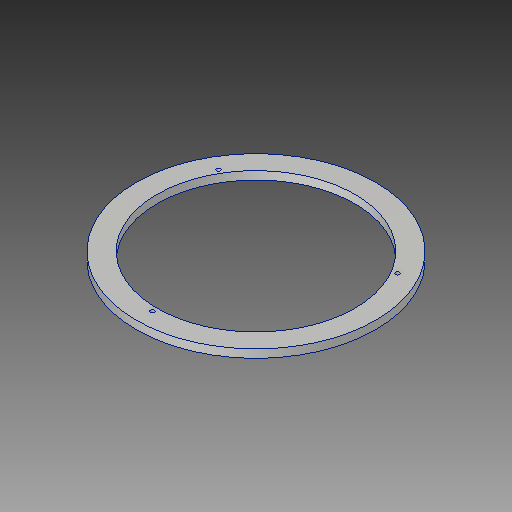
# Autodesk Inventor part: LazySusan
Saved by Autodesk Inventor 2019 (Build 230136000, 136)
## iProperties
Created: 2015-11-16
Part Number: LazySusan
Material: Aluminum 6061
Document SubType Name: Modeling
Designer: Vervaeke-Lab
Density: 2.7 g/cm^3
Appearance: Aluminum - Flat
Author: Vervaeke-Lab
Autodesk Inventor part; units mm, degrees
ref_plane "YZ Plane" through (0, 0, 0) normal (1, 0, 0) x (0, 1, 0)
ref_plane "XZ Plane" through (0, 0, 0) normal (0, 1, 0) x (-1, 0, 0)
ref_plane "XY Plane" through (0, 0, 0) normal (0, 0, 1) x (1, 0, 0)
sketch "Sketch2" plane through (0, 0, 0) normal (0, 1, 0) x (-1, 0, 0)
  circle A0 centre (0.2452, 0) radius 150
  circle A1 centre (0.2452, 0) radius 124
  point P0 (0, 0)
  dimension "d0" = 300
  dimension "d1" = 248
  constraints: 2 centre point, 1 coincident
  measures "d0" diameter of A0
  measures "d1" diameter of A1
extrude "Extrusion1" add sketch "Sketch2" along normal blind 10.2
sketch "Sketch3" plane through (-0.2452, 10.2, 0) normal (0, 1, 0) x (1, 0, 0)
  point P0 (0.2452, 0)
  point P1 (0, -130)
  point P2 (112.9511, 64.7876)
  point P3 (-112.2155, 65.2124)
  dimension "d13" = 360
  dimension "d15" = 130
  constraints: 4 other
  measures "d15" distance of point (0.245, 0) point (0, -130)
hole "Hole1" at (-0.2452, 10.2, 130) at (112.7059, 10.2, -64.7876) at (-112.4607, 10.2, -65.2124) direction (0, -1, 0) diameter 5 end through all
body "Solid1"
